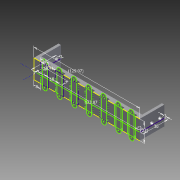
# Autodesk Inventor part: TestRack
Saved by Autodesk Inventor 2014 SP1 (Build 180222100, 222)
## iProperties
Created: 2014-06-08
Part Number: TestRack
Material: Generic
Document SubType Name: Modeling
Designer: Erin
Density: 1 g/cm^3
Appearance: Default
Author: Erin
Autodesk Inventor part; units mm, degrees
ref_plane "YZ Plane" through (0, 0, 0) normal (1, 0, 0) x (0, 1, 0)
ref_plane "XZ Plane" through (0, 0, 0) normal (0, 1, 0) x (-1, 0, 0)
ref_plane "XY Plane" through (0, 0, 0) normal (0, 0, 1) x (1, 0, 0)
sketch "Block1" plane through (0, 0, 0) normal (0, 0, 1) x (1, 0, 0)
  line L0 (113.8499, 23) -> (123.8499, 23)
  line L1 (123.8499, 23) -> (123.8499, 0)
  line L2 (123.8499, 0) -> (113.8499, 0)
  line L3 (113.8499, 0) -> (113.8499, 23)
  line L4 (118.8499, 28) -> (118.8499, 28)
  line L5 (121.8499, 25) -> (121.8499, -2)
  line L6 (118.8499, -5) -> (118.8499, -5)
  line L7 (115.8499, -2) -> (115.8499, 25)
  arc A0 (115.8499, -2) -> (118.8499, -5) centre (118.8499, -2) ccw
  arc A1 (118.8499, -5) -> (121.8499, -2) centre (118.8499, -2) ccw
  arc A2 (118.8499, 28) -> (115.8499, 25) centre (118.8499, 25) ccw
  arc A3 (121.8499, 25) -> (118.8499, 28) centre (118.8499, 25) ccw
  point P0 (118.8499, 11.5)
  dimension "d59" = 10
  dimension "d60" = 23
  dimension "d61" = 2
  dimension "d62" = 2
  dimension "d63" = 5
  dimension "d64" = 5
  dimension "d65" = 3
  measures "d59" distance of L1.end L2.end
  measures "d60" distance of L0.end L1.end
  measures "d61" distance between parallel lines of L3 L7
  measures "d62" distance between parallel lines of L1 L5
  measures "d63" distance between parallel lines of L0 L4
  measures "d64" distance between parallel lines of L2 L6
  measures "d65" radius of A0
sketch "Sketch1" plane through (0, 0, 0) normal (0, 0, 1) x (1, 0, 0)
  spline S0 degree 3 poles (2, 10) (2.0683, 9.934) (2.2049, 9.8019) (2.3976, 9.5917) (2.5801, 9.3727) (2.75, 9.1437) (2.9055, 8.9048) (3.0207, 8.6968) (3.1019, 8.525) (3.156, 8.3932) (3.2036, 8.2586) (3.224, 8.1658) (3.2342, 8.1194) knots 0 0 0 0 0.125008 0.250018 0.375026 0.500031 0.62503 0.750021 0.812527 0.87503 0.937529 1 1 1 1
  spline S1 degree 3 poles (3.2342, 8.1194) (3.2365, 8.0444) (3.24, 7.9319) (3.2585, 7.7829) (3.28, 7.6724) (3.3073, 7.5631) (3.344, 7.4566) (3.3884, 7.3531) (3.4433, 7.2547) (3.5085, 7.1628) (3.5843, 7.0792) (3.6705, 7.0064) (3.7664, 6.947) (3.8703, 6.9031) (3.9799, 6.8754) (4.0924, 6.8678) (4.2049, 6.8707) (4.3173, 6.8678) (4.4299, 6.8754) (4.5394, 6.9031) (4.6433, 6.947) (4.7393, 7.0064) (4.8255, 7.0792) (4.9012, 7.1628) (4.9665, 7.2547) (5.0214, 7.3531) (5.0657, 7.4566) (5.1024, 7.5631) (5.1297, 7.6724) (5.1513, 7.7829) (5.1697, 7.9319) (5.1732, 8.0444) (5.1755, 8.1194) knots 0 0 0 0 0.062511 0.093774 0.125034 0.156296 0.187553 0.218812 0.250072 0.281326 0.312572 0.343813 0.375055 0.40629 0.437511 0.468738 0.5 0.531262 0.562489 0.59371 0.624945 0.656187 0.687428 0.718674 0.749928 0.781188 0.812447 0.843704 0.874966 0.906226 0.937489 1 1 1 1
  spline S2 degree 3 poles (5.1755, 8.1194) (5.1858, 8.1658) (5.2062, 8.2586) (5.2538, 8.3932) (5.3078, 8.525) (5.3891, 8.6968) (5.5042, 8.9048) (5.6598, 9.1437) (5.8297, 9.3727) (6.0122, 9.5917) (6.2048, 9.8019) (6.3414, 9.934) (6.4098, 10) knots 0 0 0 0 0.062471 0.12497 0.187473 0.249979 0.37497 0.499969 0.624974 0.749982 0.874992 1 1 1 1
  line L0 (0, 10) -> (2, 10)
  line L1 (0, 3) -> (123.07, 3)
  line L2 (0, 3) -> (0, 10)
  line L3 (123.07, 3) -> (123.07, 10)
  arc A0 (2, 10) -> (0, 10) centre (1, 10) ccw
  line L4 (121.07, 10) -> (121.07, 3) construction
  arc A1 (123.07, 10) -> (121.07, 10) centre (122.07, 10) ccw
  line L5 (6.4098, 10) -> (123.07, 10)
  line L6 (2, 10) -> (6.4098, 10)
  line L7 (0, 3) -> (123.07, 3)
  line L8 (123.07, 3) -> (123.07, 0)
  line L9 (123.07, 0) -> (0, 0)
  line L10 (0, 0) -> (0, 3)
  line L11 (0, 24) -> (0, -16) construction
  line L12 (-20, 0) -> (0, 0) construction
  line L13 (0, 0) -> (-3, 0)
  line L14 (-3, 0) -> (-3, 30)
  line L15 (-3, 30) -> (0, 30)
  line L16 (0, 30) -> (0, 0)
  line L17 (123.07, 0) -> (126.07, 0)
  line L18 (126.07, 0) -> (126.07, 30)
  line L19 (126.07, 30) -> (123.07, 30)
  line L20 (123.07, 30) -> (123.07, 0)
  point P0 (2.2029, 9.7999)
  point P1 (2.3959, 9.5902)
  point P2 (2.578, 9.371)
  point P3 (2.7476, 9.1421)
  point P4 (2.9026, 8.903)
  point P5 (3.0401, 8.6534)
  point P6 (3.1008, 8.5245)
  point P7 (3.1549, 8.3927)
  point P8 (3.2007, 8.2578)
  point P9 (3.2458, 7.8947)
  point P10 (3.2597, 7.7831)
  point P11 (3.281, 7.6726)
  point P12 (3.3089, 7.5636)
  point P13 (3.3453, 7.4571)
  point P14 (3.3901, 7.354)
  point P15 (3.445, 7.2557)
  point P16 (3.5103, 7.1641)
  point P17 (3.586, 7.081)
  point P18 (3.6721, 7.0087)
  point P19 (3.7678, 6.9496)
  point P20 (3.8713, 6.9058)
  point P21 (3.9804, 6.8787)
  point P22 (4.0924, 6.8696)
  point P23 (4.2049, 6.8698)
  point P24 (4.3174, 6.8696)
  point P25 (4.4294, 6.8787)
  point P26 (4.5385, 6.9058)
  point P27 (4.642, 6.9496)
  point P28 (4.7377, 7.0087)
  point P29 (4.8237, 7.081)
  point P30 (4.8995, 7.1641)
  point P31 (4.9648, 7.2557)
  point P32 (5.0196, 7.354)
  point P33 (5.0645, 7.4571)
  point P34 (5.1009, 7.5636)
  point P35 (5.1288, 7.6726)
  point P36 (5.15, 7.7831)
  point P37 (5.164, 7.8947)
  point P38 (5.209, 8.2578)
  point P39 (5.2549, 8.3927)
  point P40 (5.309, 8.5245)
  point P41 (5.3697, 8.6534)
  point P42 (5.5071, 8.903)
  point P43 (5.6622, 9.1421)
  point P44 (5.8318, 9.371)
  point P45 (6.0139, 9.5902)
  point P46 (6.2069, 9.7999)
  dimension "d2" = 7
  dimension "d3" = 123.07
  dimension "d4" = 2
  dimension "d5" = 4.4097
  dimension "d6" = 2
  dimension "d14" = 3
  dimension "d26" = 30
  dimension "d27" = 3
  dimension "d28" = 3
  dimension "d29" = 30
  constraints: 42 end point, 7 horizontal, 7 parallel, 6 perpendicular, 4 point on circle, 3 point on line, 3 tangent, 2 centre point, 2 collinear, 2 vertical, 55 other
  measures "d2" distance between parallel lines of L1 L0
  measures "d3" distance of L1.start L1.end
  measures "d4" distance from line of L0.end L2
  measures "d5" distance of L5.start L0.end
  measures "d6" distance between parallel lines of L4 L3
  measures "d14" distance of L9.end L1.start
  measures "d26" distance of L13.end L14.end
  measures "d27" distance of L14.end L15.end
  measures "d28" distance of L18.end L19.end
  measures "d29" distance of L17.end L18.end
extrude "Extrusion2" add sketch "Sketch1" along normal blind 5 contours L6 S2 S1 S0 | S0 S1 S2 L5 L3 L1 L2 L0 | L0 A0 | A1 L5
extrude "Extrusion3" cut sketch "Sketch1" along normal blind 5 contours L6 S2 S1 S0
pattern_linear "Rectangular Pattern1" count 27 spacing 4.41 along (1, 0, 0) of "Extrusion3"
extrude "Extrusion4" add sketch "Sketch1" along normal blind 14 contours L1 L8 L9 L10
sketch "Sketch2" plane through (0, 3, 5) normal (0, 1, 0) x (1, 0, 0)
  line L0 (123.07, 0) -> (123.07, -9) projected
  line L1 (0, 0) -> (123.07, 0)
  line L2 (123.07, 0) -> (123.07, -2.8)
  line L3 (123.07, -2.8) -> (0, -2.8)
  line L4 (0, -2.8) -> (0, 0)
  line L5 (0, -9) -> (123.07, -9)
  line L6 (123.07, -9) -> (123.07, -6.2)
  line L7 (123.07, -6.2) -> (0, -6.2)
  line L8 (0, -6.2) -> (0, -9)
  point P0 (0, 5)
  dimension "d17" = 2.8
  dimension "d18" = 2.8
  constraints: 16 end point, 4 parallel, 2 horizontal, 2 perpendicular, 2 point on line
  measures "d17" distance between parallel lines of L3 L1
  measures "d18" distance between parallel lines of L5 L7
extrude "Extrusion5" add sketch "Sketch2" along normal blind 3
extrude "Extrusion6" add sketch "Sketch1" against normal blind 9 contours L1 L8 L9 L10
sketch "Sketch3" plane through (0, 3, 0) normal (0, 1, 0) x (1, 0, 0)
  line L0 (123.07, 0) -> (123.07, 9) projected
  line L1 (0, 9) -> (123.07, 9)
  line L2 (123.07, 9) -> (123.07, 6.2)
  line L3 (123.07, 6.2) -> (0, 6.2)
  line L4 (0, 6.2) -> (0, 9)
  line L5 (0, 0) -> (123.07, 0)
  line L6 (123.07, 0) -> (123.07, 2.8)
  line L7 (123.07, 2.8) -> (0, 2.8)
  line L8 (0, 2.8) -> (0, 0)
  dimension "d23" = 2.8
  dimension "d47" = 2.8
  constraints: 16 end point, 4 parallel, 2 horizontal, 2 perpendicular, 2 point on line
  measures "d23" distance of L1.end L2.end
  measures "d47" distance of L5.end L6.end
extrude "Extrusion7" add sketch "Sketch3" along normal blind 3
extrude "Extrusion8" add sketch "Sketch1" along normal blind 14 contours L2 L10 L13 L14 L15 L16 | L3 L20 L19 L18 L17 L8
extrude "Extrusion9" add sketch "Sketch1" against normal blind 9 contours L2 L10 L13 L14 L15 L16 | L3 L20 L19 L18 L17 L8
sketch "Sketch4" plane through (-3, 0, 14) normal (-1, 0, 0) x (0, 0, 1)
  line L0 (-23, 0) -> (0, 0) projected
  line L1 (-23, 30) -> (0, 30) projected
  line L2 (-11.5, 30) -> (-11.5, 0) construction
  circle A0 centre (-11.5, 25) radius 2.25
  circle A1 centre (-11.5, 15) radius 2.25
  point P0 (-14, 0)
  dimension "d34" = 4.5
  dimension "d35" = 4.5
  dimension "d36" = 5
  dimension "d38" = 15
  constraints: 3 midpoint, 2 centre point, 2 end point, 1 point on line
  measures "d34" diameter of A0
  measures "d35" diameter of A1
  measures "d36" distance from line of A0.centre L1
  measures "d38" distance from line of A1.centre L1
extrude "Extrusion10" cut sketch "Sketch4" against normal blind 4
sketch "Sketch5" plane through (126.07, 0, 14) normal (1, 0, 0) x (0, 0, -1)
  line L0 (23, 30) -> (0, 30) projected
  line L1 (23, 0) -> (0, 0) projected
  line L2 (11.5, 30) -> (11.5, 0) construction
  circle A0 centre (11.5, 25) radius 2.25
  circle A1 centre (11.5, 15) radius 2.25
  point P0 (14, 0)
  dimension "d41" = 4.5
  dimension "d42" = 4.5
  dimension "d43" = 5
  dimension "d44" = 15
  constraints: 3 midpoint, 2 centre point, 2 end point, 1 point on line
  measures "d41" diameter of A0
  measures "d42" diameter of A1
  measures "d43" distance from line of A0.centre L0
  measures "d44" distance from line of A1.centre L0
extrude "Extrusion11" cut sketch "Sketch5" against normal blind 4
sketch "Sketch6" plane through (-3, 0, -9) normal (0, -1, 0) x (1, 0, 0)
  line L0 (129.07, 0) -> (0, 0) projected
  line L1 (0, 23) -> (129.07, 23) projected
  line L2 (0, 0) -> (0, 23) projected
  line L3 (8, 23) -> (18, 23)
  line L4 (18, 23) -> (18, 0)
  line L5 (18, 0) -> (8, 0)
  line L6 (8, 0) -> (8, 23)
  line L7 (26, 23) -> (36, 23)
  line L8 (36, 23) -> (36, 0)
  line L9 (36, 0) -> (26, 0)
  line L10 (26, 0) -> (26, 23)
  line L11 (44, 23) -> (54, 23)
  line L12 (54, 23) -> (54, 0)
  line L13 (54, 0) -> (44, 0)
  line L14 (44, 0) -> (44, 23)
  line L15 (62, 23) -> (72, 23)
  line L16 (72, 23) -> (72, 0)
  line L17 (72, 0) -> (62, 0)
  line L18 (62, 0) -> (62, 23)
  line L19 (80, 23) -> (90, 23)
  line L20 (90, 23) -> (90, 0)
  line L21 (90, 0) -> (80, 0)
  line L22 (80, 0) -> (80, 23)
  line L23 (113.8499, 23) -> (123.8499, 23)
  line L24 (123.8499, 23) -> (123.8499, 0)
  line L25 (123.8499, 0) -> (113.8499, 0)
  line L26 (113.8499, 0) -> (113.8499, 23)
  line L27 (118.8499, 28) -> (118.8499, 28)
  line L28 (121.8499, 25) -> (121.8499, -2)
  line L29 (118.8499, -5) -> (118.8499, -5)
  line L30 (115.8499, -2) -> (115.8499, 25)
  arc A0 (115.8499, -2) -> (118.8499, -5) centre (118.8499, -2) ccw
  arc A1 (118.8499, -5) -> (121.8499, -2) centre (118.8499, -2) ccw
  arc A2 (118.8499, 28) -> (115.8499, 25) centre (118.8499, 25) ccw
  arc A3 (121.8499, 25) -> (118.8499, 28) centre (118.8499, 25) ccw
  line L31 (8, 23) -> (18, 23)
  line L32 (18, 23) -> (18, 0)
  line L33 (18, 0) -> (8, 0)
  line L34 (8, 0) -> (8, 23)
  line L35 (13, 28) -> (13, 28)
  line L36 (16, 25) -> (16, -2)
  line L37 (13, -5) -> (13, -5)
  line L38 (10, -2) -> (10, 25)
  arc A4 (10, -2) -> (13, -5) centre (13, -2) ccw
  arc A5 (13, -5) -> (16, -2) centre (13, -2) ccw
  arc A6 (13, 28) -> (10, 25) centre (13, 25) ccw
  arc A7 (16, 25) -> (13, 28) centre (13, 25) ccw
  line L39 (26, 23) -> (36, 23)
  line L40 (36, 23) -> (36, 0)
  line L41 (36, 0) -> (26, 0)
  line L42 (26, 0) -> (26, 23)
  line L43 (31, 28) -> (31, 28)
  line L44 (34, 25) -> (34, -2)
  line L45 (31, -5) -> (31, -5)
  line L46 (28, -2) -> (28, 25)
  arc A8 (28, -2) -> (31, -5) centre (31, -2) ccw
  arc A9 (31, -5) -> (34, -2) centre (31, -2) ccw
  arc A10 (31, 28) -> (28, 25) centre (31, 25) ccw
  arc A11 (34, 25) -> (31, 28) centre (31, 25) ccw
  line L47 (44, 23) -> (54, 23)
  line L48 (54, 23) -> (54, 0)
  line L49 (54, 0) -> (44, 0)
  line L50 (44, 0) -> (44, 23)
  line L51 (49, 28) -> (49, 28)
  line L52 (52, 25) -> (52, -2)
  line L53 (49, -5) -> (49, -5)
  line L54 (46, -2) -> (46, 25)
  arc A12 (46, -2) -> (49, -5) centre (49, -2) ccw
  arc A13 (49, -5) -> (52, -2) centre (49, -2) ccw
  arc A14 (49, 28) -> (46, 25) centre (49, 25) ccw
  arc A15 (52, 25) -> (49, 28) centre (49, 25) ccw
  line L55 (62, 23) -> (72, 23)
  line L56 (72, 23) -> (72, 0)
  line L57 (72, 0) -> (62, 0)
  line L58 (62, 0) -> (62, 23)
  line L59 (67, 28) -> (67, 28)
  line L60 (70, 25) -> (70, -2)
  line L61 (67, -5) -> (67, -5)
  line L62 (64, -2) -> (64, 25)
  arc A16 (64, -2) -> (67, -5) centre (67, -2) ccw
  arc A17 (67, -5) -> (70, -2) centre (67, -2) ccw
  arc A18 (67, 28) -> (64, 25) centre (67, 25) ccw
  arc A19 (70, 25) -> (67, 28) centre (67, 25) ccw
  line L63 (80, 23) -> (90, 23)
  line L64 (90, 23) -> (90, 0)
  line L65 (90, 0) -> (80, 0)
  line L66 (80, 0) -> (80, 23)
  line L67 (85, 28) -> (85, 28)
  line L68 (88, 25) -> (88, -2)
  line L69 (85, -5) -> (85, -5)
  line L70 (82, -2) -> (82, 25)
  arc A20 (82, -2) -> (85, -5) centre (85, -2) ccw
  arc A21 (85, -5) -> (88, -2) centre (85, -2) ccw
  arc A22 (85, 28) -> (82, 25) centre (85, 25) ccw
  arc A23 (88, 25) -> (85, 28) centre (85, 25) ccw
  line L71 (98, 23) -> (108, 23)
  line L72 (108, 23) -> (108, 0)
  line L73 (108, 0) -> (98, 0)
  line L74 (98, 0) -> (98, 23)
  line L75 (103, 28) -> (103, 28)
  line L76 (106, 25) -> (106, -2)
  line L77 (103, -5) -> (103, -5)
  line L78 (100, -2) -> (100, 25)
  arc A24 (100, -2) -> (103, -5) centre (103, -2) ccw
  arc A25 (103, -5) -> (106, -2) centre (103, -2) ccw
  arc A26 (103, 28) -> (100, 25) centre (103, 25) ccw
  arc A27 (106, 25) -> (103, 28) centre (103, 25) ccw
  point P0 (3, 9)
  dimension "d76" = 18
  dimension "d48" = 129.07
  dimension "d49" = 10
  dimension "d50" = 8
  dimension "d53" = 18
  dimension "d58" = 23
  constraints: 40 end point, 8 horizontal, 2 parallel, 2 point on line, 1 perpendicular, 32 other
  measures "d48" distance of L1.start L1.end
  measures "d49" distance between parallel lines of L4 L6
  measures "d50" distance between parallel lines of L2 L6
  measures "d53" distance of L3.start L7.start
  measures "d58" distance of L0.start L1.end
extrude "Extrusion12" cut sketch "Sketch6" against normal blind 2.5 contours L26 L1 L30 L0 | L0 L76 L1 L72 | L30 L1 L28 L0 | L0 L78 L1 L76 | L28 L1 L24 L0 | L0 L74 L1 L78 | L0 L68 L1 L20 | L0 L70 L1 L68 | L0 L22 L1 L70 | L0 L60 L1 L16 | L0 L62 L1 L60 | L0 L18 L1 L62 | L0 L52 L1 L12 | L0 L54 L1 L52 | L0 L14 L1 L54 | L0 L44 L1 L8 | L0 L46 L1 L44 | L0 L10 L1 L46 | L0 L36 L1 L4 | L0 L38 L1 L36 | L0 L6 L1 L38
extrude "Extrusion13" add sketch "Sketch6" against normal blind 0.6 contours L30 L1 L28 L0 | L0 L28 A1 A0 L30 | L76 A25 A24 L78 L0 | L0 L78 L1 L76 | L30 A2 A3 L28 L1 | L1 L78 A26 A27 L76 | L68 A21 A20 L70 L0 | L0 L70 L1 L68 | L1 L70 A22 A23 L68 | L60 A17 A16 L62 L0 | L0 L62 L1 L60 | L1 L62 A18 A19 L60 | L52 A13 A12 L54 L0 | L0 L54 L1 L52 | L1 L54 A14 A15 L52 | L44 A9 A8 L46 L0 | L0 L46 L1 L44 | L1 L46 A10 A11 L44 | L36 A5 A4 L38 L0 | L0 L38 L1 L36 | L1 L38 A6 A7 L36
equation "\"Module\" = 1.5"
equation "\"PressureAngle\" = 20deg"
equation "\"UnitProfileClearance\" = 0.25"
equation "\"UnitRoundRadius\" = 0.35"
equation "\"HeadDiameter\" = 22.44787"
equation "\"RootDiameter\" = 15.75"
equation "\"BaseDiameter\" = 18.32401"
equation "\"PitchDiameter\" = 19.5"
equation "\"FaceWidth\" = 3"
equation "\"HelixAngle\" = 0"
equation "\"UnitCorrection\" = 0"
equation "\"UnitAddendumModification\" = 0.017376"
equation "\"CircularPitch\" = 4.712389"
equation "\"UnitBacklashShift\" = 0"
equation "\"TotalToolShift\" = 0"
equation "\"IsInternal\" = 0"
equation "\"sp\" = 0.4"
body "Solid2"
